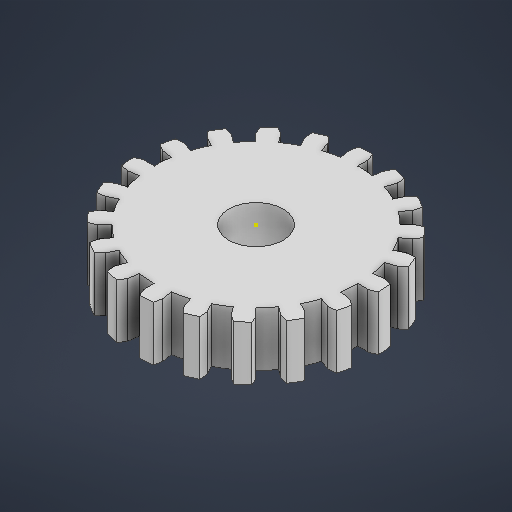
# Autodesk Inventor part: Gear1
Saved by Autodesk Inventor 2026.2 (Build 302298000, 298)
## iProperties
Created: 2025-12-18
Part Number: Gear1
Material: Generic
Document SubType Name: Modeling
Designer: Cobble
Density: 1 g/cm^3
Appearance: Default
Author: Cobble
Autodesk Inventor part; units mm, degrees
ref_plane "YZ Plane" through (0, 0, 0) normal (1, 0, 0) x (0, 1, 0)
ref_plane "XZ Plane" through (0, 0, 0) normal (0, 1, 0) x (-1, 0, 0)
ref_plane "XY Plane" through (0, 0, 0) normal (0, 0, 1) x (1, 0, 0)
sketch "Sketch1" plane through (0, 0, 0) normal (0, 0, 1) x (1, 0, 0)
  circle A0 centre (0, 0) radius 20 construction
  circle A1 centre (0, 0) radius 18.7939 construction
  circle A2 centre (0, 0) radius 22
  line L0 (0, 0) -> (0, 22)
  line L1 (0, 0) -> (22, 0) construction
  line L2 (0, 0) -> (-6.7984, 20.9232)
  line L3 (0, 0) -> (-12.9313, 17.7984)
  line L4 (0, 0) -> (-17.7984, 12.9313)
  line L5 (0, 0) -> (-20.9232, 6.7984)
  line L6 (0, 0) -> (-22, 0)
  line L7 (0, 0) -> (-20.9232, -6.7984)
  line L8 (0, 0) -> (-17.7984, -12.9313)
  line L9 (0, 0) -> (-12.9313, -17.7984)
  line L10 (0, 0) -> (-6.7984, -20.9232)
  line L11 (0, 0) -> (0, -22)
  line L12 (0, 0) -> (6.7984, -20.9232)
  line L13 (0, 0) -> (12.9313, -17.7984)
  line L14 (0, 0) -> (17.7984, -12.9313)
  line L15 (0, 0) -> (20.9232, -6.7984)
  line L16 (0, 0) -> (22, 0)
  line L17 (0, 0) -> (20.9232, 6.7984)
  line L18 (0, 0) -> (17.7984, 12.9313)
  line L19 (0, 0) -> (12.9313, 17.7984)
  line L20 (0, 0) -> (6.7984, 20.9232)
  line L21 (-5.8076, 17.874) -> (0.1679, 19.8156) construction
  line L22 (-11.0467, 15.2045) -> (-0.8806, 22.5907) construction
  line L23 (-15.2045, 11.0467) -> (-4.1254, 26.2959) construction
  line L24 (-17.874, 5.8076) -> (-10.1078, 29.7096) construction
  spline S0 degree 4 poles (0, 18.7939) (0.9486, 19.9534) (-1.4512, 25.4924) (-4.996, 27.3754) (-10.1078, 29.7096) knots 0 0 0 0 0 1 1 1 1 1 construction
  line L25 (-0.5565, 21.993) -> (-0.5565, 18.7856) construction
  line L26 (0, 20.6101) -> (-0.5565, 20.6101) construction
  line L27 (-0.2186, 21.2413) -> (-0.5565, 21.2413) construction
  line L28 (0, 0) -> (-3.1287, 19.7538)
  line L29 (0, 0) -> (20, 0) construction
  arc A3 (0, 20.6101) -> (-0.5565, 21.993) centre (-8.0106, 18.1896) ccw
  line L30 (0, 0) -> (-1.5692, 19.9383)
  line L31 (0, 0) -> (20, 0) construction
  arc A4 (-2.8908, 21.8092) -> (-3.2241, 20.3564) centre (5.0665, 19.2188) ccw
  line L32 (-3.2241, 20.3564) -> (-3.1287, 19.7538)
  circle A5 centre (0, 0) radius 18.75
  arc A6 (-6.3689, 19.6014) -> (-7.3255, 20.7446) centre (-13.2394, 14.824) ccw
  line L33 (0, 0) -> (-6.7984, 20.9232)
  arc A7 (-9.4887, 19.8485) -> (-9.3568, 18.3638) centre (-1.1205, 19.8438) ccw
  line L34 (-9.3568, 18.3638) -> (-9.0798, 17.8201)
  line L35 (0, 0) -> (-9.0798, 17.8201)
  arc A8 (-12.1143, 16.6739) -> (-13.3774, 17.4656) centre (-17.1723, 10.0072) ccw
  line L36 (0, 0) -> (-12.9313, 17.7984)
  arc A9 (-15.1578, 15.9449) -> (-14.5736, 14.5736) centre (-7.1977, 18.5264) ccw
  line L37 (-14.5736, 14.5736) -> (-14.1421, 14.1421)
  line L38 (0, 0) -> (-14.1421, 14.1421)
  arc A10 (-16.6739, 12.1143) -> (-18.1198, 12.4769) centre (-19.4242, 4.2109) ccw
  line L39 (0, 0) -> (-17.7984, 12.9313)
  arc A11 (-19.3432, 10.4805) -> (-18.3638, 9.3568) centre (-12.5704, 15.3954) ccw
  line L40 (-18.3638, 9.3568) -> (-17.8201, 9.0798)
  line L41 (0, 0) -> (-17.8201, 9.0798)
  arc A12 (-19.6014, 6.3689) -> (-21.0885, 6.2669) centre (-19.7748, -1.9976) ccw
  line L42 (0, 0) -> (-20.9232, 6.7984)
  arc A13 (-21.6351, 3.9901) -> (-20.3564, 3.2241) centre (-16.7126, 10.7574) ccw
  line L43 (-20.3564, 3.2241) -> (-19.7538, 3.1287)
  line L44 (0, 0) -> (-19.7538, 3.1287)
  arc A14 (-20.6101, 0) -> (-21.993, -0.5565) centre (-18.1896, -8.0106) ccw
  line L45 (0, 0) -> (-22, 0)
  arc A15 (-21.8092, -2.8908) -> (-20.3564, -3.2241) centre (-19.2188, 5.0665) ccw
  line L46 (-20.3564, -3.2241) -> (-19.7538, -3.1287)
  line L47 (0, 0) -> (-19.7538, -3.1287)
  arc A16 (-19.6014, -6.3689) -> (-20.7446, -7.3255) centre (-14.824, -13.2394) ccw
  line L48 (0, 0) -> (-20.9232, -6.7984)
  arc A17 (-19.8485, -9.4887) -> (-18.3638, -9.3568) centre (-19.8438, -1.1205) ccw
  line L49 (-18.3638, -9.3568) -> (-17.8201, -9.0798)
  line L50 (0, 0) -> (-17.8201, -9.0798)
  arc A18 (-16.6739, -12.1143) -> (-17.4656, -13.3774) centre (-10.0072, -17.1723) ccw
  line L51 (0, 0) -> (-17.7984, -12.9313)
  arc A19 (-15.9449, -15.1578) -> (-14.5736, -14.5736) centre (-18.5264, -7.1977) ccw
  line L52 (-14.5736, -14.5736) -> (-14.1421, -14.1421)
  line L53 (0, 0) -> (-14.1421, -14.1421)
  arc A20 (-12.1143, -16.6739) -> (-12.4769, -18.1198) centre (-4.2109, -19.4242) ccw
  line L54 (0, 0) -> (-12.9313, -17.7984)
  arc A21 (-10.4805, -19.3432) -> (-9.3568, -18.3638) centre (-15.3954, -12.5704) ccw
  line L55 (-9.3568, -18.3638) -> (-9.0798, -17.8201)
  line L56 (0, 0) -> (-9.0798, -17.8201)
  arc A22 (-6.3689, -19.6014) -> (-6.2669, -21.0885) centre (1.9976, -19.7748) ccw
  line L57 (0, 0) -> (-6.7984, -20.9232)
  arc A23 (-3.9901, -21.6351) -> (-3.2241, -20.3564) centre (-10.7574, -16.7126) ccw
  line L58 (-3.2241, -20.3564) -> (-3.1287, -19.7538)
  line L59 (0, 0) -> (-3.1287, -19.7538)
  arc A24 (0, -20.6101) -> (0.5565, -21.993) centre (8.0106, -18.1896) ccw
  line L60 (0, 0) -> (0, -22)
  arc A25 (2.8908, -21.8092) -> (3.2241, -20.3564) centre (-5.0665, -19.2188) ccw
  line L61 (3.2241, -20.3564) -> (3.1287, -19.7538)
  line L62 (0, 0) -> (3.1287, -19.7538)
  arc A26 (6.3689, -19.6014) -> (7.3255, -20.7446) centre (13.2394, -14.824) ccw
  line L63 (0, 0) -> (6.7984, -20.9232)
  arc A27 (9.4887, -19.8485) -> (9.3568, -18.3638) centre (1.1205, -19.8438) ccw
  line L64 (9.3568, -18.3638) -> (9.0798, -17.8201)
  line L65 (0, 0) -> (9.0798, -17.8201)
  arc A28 (12.1143, -16.6739) -> (13.3774, -17.4656) centre (17.1723, -10.0072) ccw
  line L66 (0, 0) -> (12.9313, -17.7984)
  arc A29 (15.1578, -15.9449) -> (14.5736, -14.5736) centre (7.1977, -18.5264) ccw
  line L67 (14.5736, -14.5736) -> (14.1421, -14.1421)
  line L68 (0, 0) -> (14.1421, -14.1421)
  arc A30 (16.6739, -12.1143) -> (18.1198, -12.4769) centre (19.4242, -4.2109) ccw
  line L69 (0, 0) -> (17.7984, -12.9313)
  arc A31 (19.3432, -10.4805) -> (18.3638, -9.3568) centre (12.5704, -15.3954) ccw
  line L70 (18.3638, -9.3568) -> (17.8201, -9.0798)
  line L71 (0, 0) -> (17.8201, -9.0798)
  arc A32 (19.6014, -6.3689) -> (21.0885, -6.2669) centre (19.7748, 1.9976) ccw
  line L72 (0, 0) -> (20.9232, -6.7984)
  arc A33 (21.6351, -3.9901) -> (20.3564, -3.2241) centre (16.7126, -10.7574) ccw
  line L73 (20.3564, -3.2241) -> (19.7538, -3.1287)
  line L74 (0, 0) -> (19.7538, -3.1287)
  arc A34 (20.6101, 0) -> (21.993, 0.5565) centre (18.1896, 8.0106) ccw
  line L75 (0, 0) -> (22, 0)
  arc A35 (21.8092, 2.8908) -> (20.3564, 3.2241) centre (19.2188, -5.0665) ccw
  line L76 (20.3564, 3.2241) -> (19.7538, 3.1287)
  line L77 (0, 0) -> (19.7538, 3.1287)
  arc A36 (19.6014, 6.3689) -> (20.7446, 7.3255) centre (14.824, 13.2394) ccw
  line L78 (0, 0) -> (20.9232, 6.7984)
  arc A37 (19.8485, 9.4887) -> (18.3638, 9.3568) centre (19.8438, 1.1205) ccw
  line L79 (18.3638, 9.3568) -> (17.8201, 9.0798)
  line L80 (0, 0) -> (17.8201, 9.0798)
  arc A38 (16.6739, 12.1143) -> (17.4656, 13.3774) centre (10.0072, 17.1723) ccw
  line L81 (0, 0) -> (17.7984, 12.9313)
  arc A39 (15.9449, 15.1578) -> (14.5736, 14.5736) centre (18.5264, 7.1977) ccw
  line L82 (14.5736, 14.5736) -> (14.1421, 14.1421)
  line L83 (0, 0) -> (14.1421, 14.1421)
  arc A40 (12.1143, 16.6739) -> (12.4769, 18.1198) centre (4.2109, 19.4242) ccw
  line L84 (0, 0) -> (12.9313, 17.7984)
  arc A41 (10.4805, 19.3432) -> (9.3568, 18.3638) centre (15.3954, 12.5704) ccw
  line L85 (9.3568, 18.3638) -> (9.0798, 17.8201)
  line L86 (0, 0) -> (9.0798, 17.8201)
  arc A42 (6.3689, 19.6014) -> (6.2669, 21.0885) centre (-1.9976, 19.7748) ccw
  line L87 (0, 0) -> (6.7984, 20.9232)
  arc A43 (3.9901, 21.6351) -> (3.2241, 20.3564) centre (10.7574, 16.7126) ccw
  line L88 (3.2241, 20.3564) -> (3.1287, 19.7538)
  line L89 (0, 0) -> (3.1287, 19.7538)
  point P0 (-7.3255, 20.7446)
  point P1 (-6.7718, 20.1341)
  point P2 (-13.3774, 17.4656)
  point P3 (-12.6621, 17.0561)
  point P4 (-18.1198, 12.4769)
  point P5 (-17.313, 12.3085)
  point P6 (-21.0885, 6.2669)
  point P7 (-20.2692, 6.3561)
  point P8 (-21.993, -0.5565)
  point P9 (-21.2413, -0.2186)
  point P10 (-18.7939, 0)
  point P11 (-20.7446, -7.3255)
  point P12 (-20.1341, -6.7718)
  point P13 (-17.874, -5.8076)
  point P14 (-17.4656, -13.3774)
  point P15 (-17.0561, -12.6621)
  point P16 (-15.2045, -11.0467)
  point P17 (-12.4769, -18.1198)
  point P18 (-12.3085, -17.313)
  point P19 (-11.0467, -15.2045)
  point P20 (-6.2669, -21.0885)
  point P21 (-6.3561, -20.2692)
  point P22 (-5.8076, -17.874)
  point P23 (0.5565, -21.993)
  point P24 (0.2186, -21.2413)
  point P25 (0, -18.7939)
  point P26 (7.3255, -20.7446)
  point P27 (6.7718, -20.1341)
  point P28 (5.8076, -17.874)
  point P29 (13.3774, -17.4656)
  point P30 (12.6621, -17.0561)
  point P31 (11.0467, -15.2045)
  point P32 (18.1198, -12.4769)
  point P33 (17.313, -12.3085)
  point P34 (15.2045, -11.0467)
  point P35 (21.0885, -6.2669)
  point P36 (20.2692, -6.3561)
  point P37 (17.874, -5.8076)
  point P38 (21.993, 0.5565)
  point P39 (21.2413, 0.2186)
  point P40 (18.7939, 0)
  point P41 (20.7446, 7.3255)
  point P42 (20.1341, 6.7718)
  point P43 (17.874, 5.8076)
  point P44 (17.4656, 13.3774)
  point P45 (17.0561, 12.6621)
  point P46 (15.2045, 11.0467)
  point P47 (12.4769, 18.1198)
  point P48 (12.3085, 17.313)
  point P49 (11.0467, 15.2045)
  point P50 (6.2669, 21.0885)
  point P51 (6.3561, 20.2692)
  point P52 (5.8076, 17.874)
  point P53 (-5.7941, 17.8323)
  point P54 (-6.3689, 19.6014)
  point P55 (-7.3255, 20.7446)
  point P56 (-8.5123, 16.7064)
  point P57 (-11.021, 15.1691)
  point P58 (-12.1143, 16.6739)
  point P59 (-13.3774, 17.4656)
  point P60 (-15.1578, 15.9449)
  point P61 (-13.2583, 13.2583)
  point P62 (-15.1691, 11.021)
  point P63 (-16.6739, 12.1143)
  point P64 (-18.1198, 12.4769)
  point P65 (-19.3432, 10.4805)
  point P66 (-16.7064, 8.5123)
  point P67 (-17.8323, 5.7941)
  point P68 (-19.6014, 6.3689)
  point P69 (-21.0885, 6.2669)
  point P70 (-21.6351, 3.9901)
  point P71 (-18.5192, 2.9331)
  point P72 (-18.75, 0)
  point P73 (-20.6101, 0)
  point P74 (-21.993, -0.5565)
  point P75 (-21.8092, -2.8908)
  point P76 (-18.5192, -2.9331)
  point P77 (-17.8323, -5.7941)
  point P78 (-19.6014, -6.3689)
  point P79 (-20.7446, -7.3255)
  point P80 (-19.8485, -9.4887)
  point P81 (-16.7064, -8.5123)
  point P82 (-15.1691, -11.021)
  point P83 (-16.6739, -12.1143)
  point P84 (-17.4656, -13.3774)
  point P85 (-15.9449, -15.1578)
  point P86 (-13.2583, -13.2583)
  point P87 (-11.021, -15.1691)
  point P88 (-12.1143, -16.6739)
  point P89 (-12.4769, -18.1198)
  point P90 (-8.5123, -16.7064)
  point P91 (-5.7941, -17.8323)
  point P92 (-6.3689, -19.6014)
  point P93 (-6.2669, -21.0885)
  point P94 (-3.9901, -21.6351)
  point P95 (-2.9331, -18.5192)
  point P96 (0, -18.75)
  point P97 (0, -20.6101)
  point P98 (0.5565, -21.993)
  point P99 (2.8908, -21.8092)
  point P100 (2.9331, -18.5192)
  point P101 (5.7941, -17.8323)
  point P102 (6.3689, -19.6014)
  point P103 (7.3255, -20.7446)
  point P104 (9.4887, -19.8485)
  point P105 (8.5123, -16.7064)
  point P106 (11.021, -15.1691)
  point P107 (12.1143, -16.6739)
  point P108 (13.3774, -17.4656)
  point P109 (15.1578, -15.9449)
  point P110 (13.2583, -13.2583)
  point P111 (15.1691, -11.021)
  point P112 (16.6739, -12.1143)
  point P113 (18.1198, -12.4769)
  point P114 (16.7064, -8.5123)
  point P115 (17.8323, -5.7941)
  point P116 (19.6014, -6.3689)
  point P117 (21.0885, -6.2669)
  point P118 (21.6351, -3.9901)
  point P119 (18.5192, -2.9331)
  point P120 (18.75, 0)
  point P121 (20.6101, 0)
  point P122 (21.993, 0.5565)
  point P123 (21.8092, 2.8908)
  point P124 (18.5192, 2.9331)
  point P125 (17.8323, 5.7941)
  point P126 (19.6014, 6.3689)
  point P127 (20.7446, 7.3255)
  point P128 (19.8485, 9.4887)
  point P129 (16.7064, 8.5123)
  point P130 (15.1691, 11.021)
  point P131 (17.4656, 13.3774)
  point P132 (15.9449, 15.1578)
  point P133 (13.2583, 13.2583)
  point P134 (11.021, 15.1691)
  point P135 (12.4769, 18.1198)
  point P136 (8.5123, 16.7064)
  point P137 (5.7941, 17.8323)
  point P138 (6.3689, 19.6014)
  point P139 (6.2669, 21.0885)
  point P140 (3.9901, 21.6351)
  point P141 (2.9331, 18.5192)
  point P142 (0, 18.75)
  point P143 (-2.8908, 21.8092)
  point P144 (-2.9331, 18.5192)
  dimension "d2" = 44
  dimension "d15" = 37.5
  dimension "d0" = 40
  dimension "d1" = 37.5877
  dimension "d6" = 360
  dimension "d9" = 6.283
  dimension "d10" = 12.566
  dimension "d11" = 18.849
  dimension "d12" = 25.132
  dimension "d13" = 99
  dimension "d14" = 94.5
  dimension "d18" = 360
  constraints: 180 end point, 128 point on circle, 46 point on line, 42 centre point, 6 perpendicular, 4 coincident, 4 horizontal, 4 tangent, 3 symmetric about line, 2 equal length, 2 vertical, 438 other
  measures "d0" diameter of A0
  measures "d1" diameter of A1
  measures "d9" distance of L21.start L21.end
  measures "d10" distance of L22.start L22.end
  measures "d11" distance of L23.start L23.end
  measures "d12" distance of L24.start L24.end
  measures "d13" angle of L29 L28
  measures "d14" angle of L31 L30
extrude "Extrusion1" add sketch "Sketch1" along normal blind 10 contours A34 L16 A5 L77 L76 A35 A2 | A2 A32 L15 A5 L74 L73 A33 | A5 L74 L16 | L16 L77 A5 | L30 A5 L0 | L35 A5 L2 | L38 A5 L3 | L41 A5 L4 | L44 A5 L5 | L47 A5 L6 | L50 A5 L7 | L53 A5 L8 | L56 A5 L9 | L59 A5 L10 | L62 A5 L11 | L65 A5 L12 | L68 A5 L13 | L71 A5 L14 | L74 A5 L15 | L80 A5 L17 | L83 A5 L18 | L86 A5 L19 | L89 A5 L20 | L2 A5 L28 | L28 A5 L30 | L3 A5 L35 | L4 A5 L38 | L5 A5 L41 | L6 A5 L44 | L7 A5 L47 | L8 A5 L50 | L9 A5 L53 | L10 A5 L56 | L11 A5 L59 | L12 A5 L62 | L13 A5 L65 | L14 A5 L68 | L15 A5 L71 | L17 A5 L77 | L18 A5 L80 | L19 A5 L83 | L20 A5 L86 | L0 A5 L89 | A36 L17 A5 L80 L79 A37 A2 | A2 A30 L14 A5 L71 L70 A31 | A5 L28 L32 A4 A2 A3 L0 | A5 L35 L34 A7 A2 A6 L2 | A5 L38 L37 A9 A2 A8 L3 | A5 L41 L40 A11 A2 A10 L4 | A5 L44 L43 A13 A2 A12 L5 | A5 L47 L46 A15 A2 A14 L6 | A5 L50 L49 A17 A2 A16 L7 | A5 L53 L52 A19 A2 A18 L8 | A5 L56 L55 A21 A2 A20 L9 | A5 L59 L58 A23 A2 A22 L10 | A5 L62 L61 A25 A2 A24 L11 | A5 L65 L64 A27 A2 A26 L12 | A5 L68 L67 A29 A2 A28 L13 | A5 L83 L82 A39 A2 A38 L18 | A5 L86 L85 A41 A2 A40 L19 | A5 L89 L88 A43 A2 A42 L20
sketch "Sketch2" plane through (0, 0, 10) normal (0, 0, 1) x (1, 0, 0)
  point P0 (0, 0)
sketch "Sketch3" plane through (0, 0, 10) normal (0, 0, 1) x (1, 0, 0)
  circle A0 centre (0, 0) radius 5
  dimension "d22" = 10
  constraints: 1 centre point, 1 coincident
  measures "d22" diameter of A0
extrude "Extrusion2" cut sketch "Sketch3" against normal blind 10
body "Solid1"
